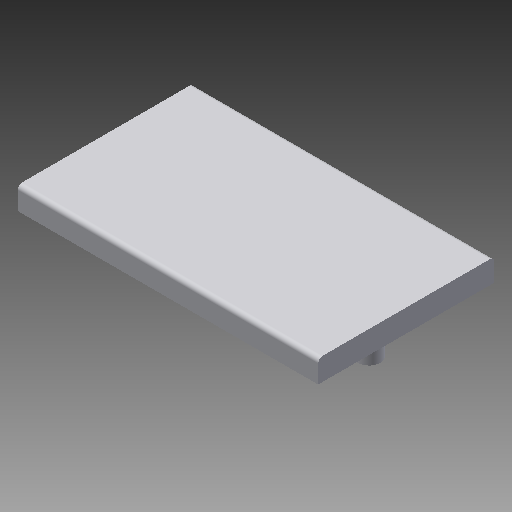
# Autodesk Inventor part: ESG 8x13.5 1912130000
Saved by Autodesk Inventor 2019.3 (Build 233278000, 278)
## iProperties
Category: PARTsolutions
Company: WEIDMUELLER
Created: 2018-11-15
Part Number: ESG 8x13.5 1912130000
Material: Generic
Catalog Web Link: www.cadenas.de
Description: ESG 8x13.5-Electronics housings
Vendor: WEIDMUELLER
Document SubType Name: Modeling
Designer: psadmin
Manufacturer: WEIDMUELLER
Mass: 0.106182 g
Surface Area: 2.58044 cm^2
Volume: 0.106182 cm^3
Density: 1 g/cm^3
Appearance: PSOLRGB-255-255-255
PSOL_IDENT_0: {$CADENAS_DATA\23d-libs\weidmueller\elektronikgehaeuse\einbaugehaeuse\ch20m\zubehoer\esg_8x13-5.prj}
PSOL_IDENT_1: ,186 {VTYP=3D},{NB=ESG 8x13.5 1912130000},{LINA=ESG 8x13.5 1912130000},{NN=ESG 8x13.5},{DATE=31.03.2
PSOL_IDENT_2: 017 09:22:39},{GEOMDATE=25.06.2010 00:00:00},{VERSION=},{LINEID=10},{WBVAR=},{WBNUMERIC=}  {NB=ESG 8
PSOL_IDENT_3: x13.5 1912130000},{LINA=ESG 8x13.5 1912130000},{KT=DUMMY},{BEST=1912130000},{BZ=ESG 8x13.5},{FCODE=1
PSOL_IDENT_4: .00,1.00,1.00,0.00}
NN: ESG 8x13.5
NT: Electronics housings
NB: ESG 8x13.5 1912130000
NBSYN: $BZ. $BEST.
LINA: ESG 8x13.5 1912130000
BEST: 1912130000
BZ: ESG 8x13.5
SUPPLIER: WEIDMUELLER
ARTICLENO: ESG 8x13.5 1912130000
BOMINFO: ESG 8x13.5 1912130000
CREATOR: CADENAS GmbH
Title: ESG 8x13.5 1912130000
Author: Cadenas PARTsolutions
Comments: Electronics housings
Autodesk Inventor part; units mm, degrees
sketch "Sketch_1" plane through (0, 0, 0) normal (1, 0, 0) x (0, 1, 0)
  line L0 (0.8, 3.9) -> (0, 3.9)
  line L1 (0, 3.9) -> (0, -3.9)
  line L2 (0, -3.9) -> (0.8, -3.9)
  arc A0 (0.8, -3.9) -> (1, -3.7) centre (0.8, -3.7) ccw
  line L3 (1, -3.7) -> (1, 3.7)
  arc A1 (1, 3.7) -> (0.8, 3.9) centre (0.8, 3.7) ccw
  constraints: 8 end point, 4 point on circle, 2 centre point
extrude "Extrusion1" add sketch "Sketch_1" along normal mid plane 13.3
sketch "Sketch_2" plane through (0, 0, 0) normal (0, 0, 1) x (1, 0, 0)
  line L0 (5, -1.7) -> (5, 0)
  line L1 (5, 0) -> (5.5, 0)
  line L2 (5.5, 0) -> (5.5, -1.7)
  line L3 (5.5, -1.7) -> (5, -1.7)
  line L4 (5, -1.7) -> (5, 0)
  constraints: 10 end point
revolve "Revolution1" add sketch "Sketch_2" angle 360 about axis through (5, -1.7, 0) along (0, -1, 0)
sketch "Sketch_3" plane through (0, 0, 0) normal (0, 0, 1) x (1, 0, 0)
  line L0 (-5, -1.7) -> (-5, 0)
  line L1 (-5, 0) -> (-4.5, 0)
  line L2 (-4.5, 0) -> (-4.5, -1.7)
  line L3 (-4.5, -1.7) -> (-5, -1.7)
  line L4 (-5, -1.7) -> (-5, 0)
  constraints: 10 end point
revolve "Revolution2" add sketch "Sketch_3" angle 360 about axis through (-5, -1.7, 0) along (0, -1, 0)
ref_plane "mitCover_XY" through (0, 0, 0) normal (0, 1, 0) x (1, 0, 0)
ref_plane "mitCover_YZ" through (0, 0, 0) normal (1, 0, 0) x (0, 0, -1)
ref_plane "mitCover_ZX" through (0, 0, 0) normal (0, 0, -1) x (0, 1, 0)
body "Solid1"
